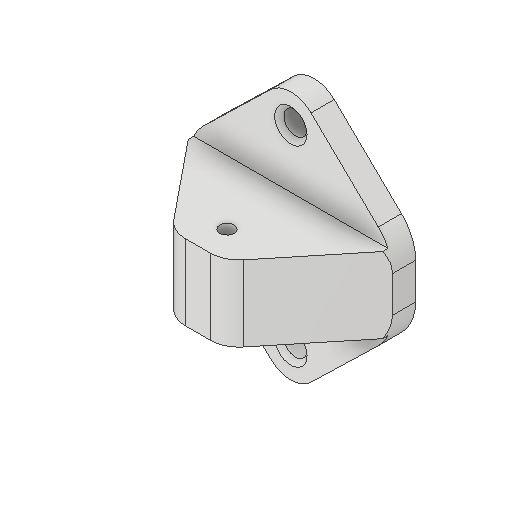
# Autodesk Inventor part: 3DP_PLA_Part_Detector_Base
Saved by Autodesk Inventor 2025 (Build 290162010, 162A)
## iProperties
Created: 2018-06-15
Part Number: 3DP_PLA_Part_Detector_Base
Material: ABS Plastic
Document SubType Name: Modeling
Designer: Andrzej
Density: 1.06 g/cm^3
Appearance: Smooth - White
Author: Andrzej
Autodesk Inventor part; units mm, degrees
ref_plane "YZ Plane" through (0, 0, 0) normal (1, 0, 0) x (0, 1, 0)
ref_plane "XZ Plane" through (0, 0, 0) normal (0, 1, 0) x (-1, 0, 0)
ref_plane "XY Plane" through (0, 0, 0) normal (0, 0, 1) x (1, 0, 0)
sketch "Sketch1" plane through (0, 0, 0) normal (0, 0, 1) x (1, 0, 0)
  line L0 (-17.5, 6.5) -> (17.5, 6.5)
  line L1 (17.5, 6.5) -> (17.5, -6.5)
  line L2 (17.5, -6.5) -> (-17.5, -6.5)
  line L3 (-17.5, -6.5) -> (-17.5, 6.5)
  circle A0 centre (0, 16.5) radius 5
  line L4 (-17.5, 6.5) -> (-3.4801, 20.0901)
  line L5 (17.5, 6.5) -> (3.4801, 20.0901)
  circle A1 centre (0, 16.5) radius 2
  point P0 (0, 0)
  dimension "d0" = 35
  dimension "d1" = 13
  dimension "d5" = 17.5
  dimension "d6" = 6.5
  dimension "d13" = 10
  dimension "d14" = 10
  dimension "d15" = 4
  constraints: 12 end point, 2 centre point, 2 parallel, 2 point on circle, 2 tangent, 1 coincident, 1 horizontal, 1 perpendicular
  measures "d0" distance of L1.end L2.end
  measures "d1" distance of L0.end L1.end
  measures "d5" distance from line of L3 point (0, 0)
  measures "d6" distance from line of L0 point (0, 0)
  measures "d13" diameter of A0
  measures "d14" distance from line of L0 A0.centre
  measures "d15" diameter of A1
extrude "Extrusion1" add sketch "Sketch1" along normal blind 20 contours L0 L1 L2 L3
extrude "Extrusion3" add sketch "Sketch1" along normal blind 4 contours L4 A0 L5 L0 | A0
mirror "Mirror3" about plane through (0, 0, 0) normal (0, 1, 0) of "Extrusion3"
chamfer "Chamfer1" distance 13 distance2 16 1 edges at (17.5, 0, 20) measured on face at (17, 0, 20)
chamfer "Chamfer2" distance 13 distance2 16 1 edges at (-17.5, 0, 20) measured on face at (-17, 0, 20)
sketch "Sketch2" plane through (-17.5, -6.5, 4) normal (0, -1, 0) x (1, 0, 0)
  line L0 (0, 0) -> (13, 16) projected
  line L1 (0, 0) -> (35, 0) projected
  line L2 (22, 16) -> (35, 0) projected
  line L3 (13, 16) -> (22, 16) projected
  point P0 (17.5, -4)
  point P1 (17.5, 11)
  dimension "d24" = 35
  dimension "d25" = 17.5
  dimension "d26" = 5
  measures "d24" distance of L1.end L0.start
  measures "d25" horizontal distance of L0.start point (17.5, 11)
  measures "d26" distance from line of point (17.5, 11) L3
hole "Hole1" at (0, -6.5, 15) direction (0, 1, 0) diameter 2.5 end through all
fillet "Fillet1" radius 5 2 edges at (-4.5, 0, 20) (4.5, 0, 20)
fillet "Fillet2" radius 8 4 edges at (-17.5, -6.5, 2) (-17.5, 6.5, 2) (17.5, -6.5, 2) (17.5, 6.5, 2)
chamfer "Chamfer3" distance 0.8 angle 45 2 edges at (-2, -16.5, 4) (-2, 16.5, 4)
equation "\"d5\" = 0.5 * d0"
equation "\"d6\" = 0.5 * d1"
equation "\"d25\" = 0.5 * d24"
body "Solid1"
